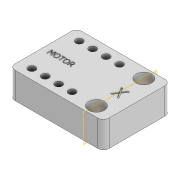
# Autodesk Inventor part: intake motor mount to xrail fixed position
Saved by Autodesk Inventor 2020 (Build 240168000, 168)
## iProperties
Created: 2020-01-10
Part Number: intake motor mount to xrail fixed position
Material: Generic
Document SubType Name: Modeling
Designer: ball
Density: 1 g/cm^3
Appearance: Default
Author: ball
Autodesk Inventor part; units mm, degrees
ref_plane "XZ Plane" through (0, 0, 0) normal (0, 1, 0) x (-1, 0, 0)
ref_plane "XY Plane" through (0, 0, 0) normal (0, 0, 1) x (1, 0, 0)
sketch "Sketch1" plane through (0, 0, 0) normal (0, 1, 0) x (-1, 0, 0)
  line L0 (-9.525, 19.05) -> (43.815, 19.05)
  line L1 (43.815, 19.05) -> (43.815, -19.05)
  line L2 (43.815, -19.05) -> (-9.525, -19.05)
  line L3 (-9.525, -19.05) -> (-9.525, 19.05)
  point P0 (0, 0)
  dimension "d0" = 53.34
  dimension "d1" = 38.1
  dimension "d3" = 9.525
  dimension "d4" = 19.05
  constraints: 8 end point, 2 parallel, 1 horizontal, 1 perpendicular
  measures "d0" distance of L1.end L2.end
  measures "d1" distance of L0.end L1.end
  measures "d3" distance from line of L3 point (0, 0)
  measures "d4" distance from line of L0 point (0, 0)
extrude "Extrusion1" add sketch "Sketch1" along normal blind 14.986
sketch "Sketch2" plane through (0, 14.986, 0) normal (0, 1, 0) x (1, 0, 0)
  line L0 (9.525, -19.05) -> (9.525, 19.05) projected
  point P0 (0, 0)
  point P1 (0, -13.4747)
  point P2 (0, 13.4747)
  dimension "d7" = 26.9494
  dimension "d9" = 9.525
  dimension "d10" = 9.525
  dimension "d11" = 13.4747
  measures "d7" distance of point (0, 13.475) point (0, -13.475)
  measures "d9" distance from line of L0 point (0, -13.475)
  measures "d10" distance from line of L0 point (0, 13.475)
  measures "d11" distance of point (0, -13.475) point (0, 0)
hole "Hole1" at (0, 14.986, 13.4747) at (0, 14.986, -13.4747) direction (0, -1, 0) diameter 4.064 end through all counterbore diameter 8.89 counterbore depth 9.0424
fillet "Fillet1" radius 3.175 4 edges at (9.525, 7.493, 19.05) (9.525, 7.493, -19.05) (-43.815, 7.493, 19.05) (-43.815, 7.493, -19.05)
sketch "Sketch5" plane through (0, 0, 0) normal (0, -1, 0) x (1, 0, 0)
  line L0 (-43.815, -15.875) -> (-43.815, 15.875) projected
  line L1 (-40.64, 19.05) -> (6.35, 19.05) projected
  line L2 (6.35, -19.05) -> (-40.64, -19.05) projected
  circle A0 centre (0, 13.4747) radius 2.032 projected
  circle A1 centre (0, -13.4747) radius 2.032 projected
  point P0 (0, 0)
  point P1 (-36.703, 13.4747)
  point P2 (-36.703, -13.4747)
  point P3 (-29.083, 13.4747)
  point P4 (-29.083, -13.4747)
  point P5 (-21.463, 13.4747)
  point P6 (-21.463, -13.4747)
  point P7 (-13.843, 13.4747)
  point P8 (-13.843, -13.4747)
  dimension "d46" = 36.703
  dimension "d47" = 36.703
  dimension "d54" = 7.62
  dimension "d59" = 26.9494
  dimension "d60" = 5.5753
  dimension "d61" = 5.5753
  constraints: 1 horizontal, 6 other
  measures "d46" distance of point (-36.703, 13.475) A0.centre
  measures "d47" distance of point (-36.703, -13.475) A1.centre
  measures "d54" distance of point (-36.703, 13.475) point (-29.083, 13.475)
  measures "d59" distance of point (-36.703, -13.475) point (-36.703, 13.475)
  measures "d60" distance from line of L1 point (-36.703, 13.475)
  measures "d61" distance from line of L2 point (-36.703, -13.475)
hole "Hole2" at (-36.703, 0, 13.4747) at (-36.703, 0, -13.4747) at (-29.083, 0, 13.4747) at (-21.463, 0, 13.4747) at (-13.843, 0, 13.4747) at (-29.083, 0, -13.4747) at (-21.463, 0, -13.4747) at (-13.843, 0, -13.4747) direction (0, 1, 0) diameter 4.064 end through all counterbore diameter 8.89 counterbore depth 6.35
sketch "Sketch6" plane through (0, 14.986, 0) normal (0, 1, 0) x (1, 0, 0)
  line L0 (-3.6028, 5.8754) -> (4.1571, 5.8754) construction
  line L1 (4.1571, 5.8754) -> (4.1571, -6.6514) construction
  line L2 (4.1571, -6.6514) -> (-3.6028, -6.6514) construction
  line L3 (-3.6028, -6.6514) -> (-3.6028, 5.8754) construction
  line L4 (-37.8576, 8.3143) -> (-28.9891, 8.3143) construction
  line L5 (-28.9891, 8.3143) -> (-28.9891, -8.4251) construction
  line L6 (-28.9891, -8.4251) -> (-37.8576, -8.4251) construction
  line L7 (-37.8576, -8.4251) -> (-37.8576, 8.3143) construction
  line L8 (-37.6075, -1.5794) -> (-38.0126, -1.5794)
  line L9 (-38.0126, -1.5794) -> (-38.0126, 1.0462)
  line L10 (-38.0126, 1.0462) -> (-38.808, -0.7396)
  line L11 (-38.808, -0.7396) -> (-39.055, -0.7396)
  line L12 (-39.055, -0.7396) -> (-39.8429, 1.0462)
  line L13 (-39.8429, 1.0462) -> (-39.8429, -1.5794)
  line L14 (-39.8429, -1.5794) -> (-40.2208, -1.5794)
  line L15 (-40.2208, -1.5794) -> (-40.2208, 1.4686)
  line L16 (-40.2208, 1.4686) -> (-39.6675, 1.4686)
  line L17 (-39.6675, 1.4686) -> (-38.9068, -0.2283)
  line L18 (-38.9068, -0.2283) -> (-38.1707, 1.4686)
  line L19 (-38.1707, 1.4686) -> (-37.6075, 1.4686)
  line L20 (-37.6075, 1.4686) -> (-37.6075, -1.5794)
  spline S0 degree 2 poles (-34.8337, 1.1203) (-34.6608, 0.9178) (-34.4682, 0.325) (-34.4682, -0.0554) knots 0 0 0 1 2 2 2
  spline S1 degree 2 poles (-34.4682, -0.0554) (-34.4682, -0.4259) (-34.6559, -1.0261) (-34.8337, -1.2287) knots 0 0 0 1 2 2 2
  spline S2 degree 2 poles (-34.8337, -1.2287) (-35.0214, -1.4411) (-35.5179, -1.6436) (-35.8168, -1.6436) knots 0 0 0 1 2 2 2
  spline S3 degree 2 poles (-35.8168, -1.6436) (-36.1255, -1.6436) (-36.6195, -1.4337) (-36.7999, -1.2287) knots 0 0 0 1 2 2 2
  spline S4 degree 2 poles (-36.7999, -1.2287) (-36.9752, -1.0261) (-37.1629, -0.4309) (-37.1629, -0.0554) knots 0 0 0 1 2 2 2
  spline S5 degree 2 poles (-37.1629, -0.0554) (-37.1629, 0.3274) (-36.9728, 0.9103) (-36.7974, 1.1203) knots 0 0 0 1 2 2 2
  spline S6 degree 2 poles (-36.7974, 1.1203) (-36.6195, 1.3228) (-36.1231, 1.5328) (-35.8168, 1.5328) knots 0 0 0 1 2 2 2
  spline S7 degree 2 poles (-35.8168, 1.5328) (-35.5056, 1.5328) (-35.0066, 1.3154) (-34.8337, 1.1203) knots 0 0 0 1 2 2 2
  spline S8 degree 2 poles (-34.8905, -0.0554) (-34.8905, 0.2459) (-35.0214, 0.7127) (-35.14, 0.8659) knots 0 0 0 1 2 2 2
  spline S9 degree 2 poles (-35.14, 0.8659) (-35.261, 1.024) (-35.6019, 1.182) (-35.8143, 1.182) knots 0 0 0 1 2 2 2
  spline S10 degree 2 poles (-35.8143, 1.182) (-36.0341, 1.182) (-36.3651, 1.0289) (-36.4911, 0.8659) knots 0 0 0 1 2 2 2
  spline S11 degree 2 poles (-36.4911, 0.8659) (-36.6121, 0.7103) (-36.7406, 0.241) (-36.7406, -0.0554) knots 0 0 0 1 2 2 2
  spline S12 degree 2 poles (-36.7406, -0.0554) (-36.7406, -0.6556) (-36.2367, -1.2929) (-35.8143, -1.2929) knots 0 0 0 1 2 2 2
  spline S13 degree 2 poles (-35.8143, -1.2929) (-35.3919, -1.2929) (-34.8905, -0.6556) (-34.8905, -0.0554) knots 0 0 0 1 2 2 2
  line L21 (-33.3122, -1.5794) -> (-33.3122, 1.1079)
  line L22 (-33.3122, 1.1079) -> (-34.3348, 1.1079)
  line L23 (-34.3348, 1.1079) -> (-34.3348, 1.4686)
  line L24 (-34.3348, 1.4686) -> (-31.8845, 1.4686)
  line L25 (-31.8845, 1.4686) -> (-31.8845, 1.1079)
  line L26 (-31.8845, 1.1079) -> (-32.9071, 1.1079)
  line L27 (-32.9071, 1.1079) -> (-32.9071, -1.5794)
  line L28 (-32.9071, -1.5794) -> (-33.3122, -1.5794)
  spline S14 degree 2 poles (-29.4194, 1.1203) (-29.2465, 0.9178) (-29.0539, 0.325) (-29.0539, -0.0554) knots 0 0 0 1 2 2 2
  spline S15 degree 2 poles (-29.0539, -0.0554) (-29.0539, -0.4259) (-29.2416, -1.0261) (-29.4194, -1.2287) knots 0 0 0 1 2 2 2
  spline S16 degree 2 poles (-29.4194, -1.2287) (-29.6072, -1.4411) (-30.1036, -1.6436) (-30.4025, -1.6436) knots 0 0 0 1 2 2 2
  spline S17 degree 2 poles (-30.4025, -1.6436) (-30.7113, -1.6436) (-31.2053, -1.4337) (-31.3856, -1.2287) knots 0 0 0 1 2 2 2
  spline S18 degree 2 poles (-31.3856, -1.2287) (-31.5609, -1.0261) (-31.7487, -0.4309) (-31.7487, -0.0554) knots 0 0 0 1 2 2 2
  spline S19 degree 2 poles (-31.7487, -0.0554) (-31.7487, 0.3274) (-31.5585, 0.9103) (-31.3831, 1.1203) knots 0 0 0 1 2 2 2
  spline S20 degree 2 poles (-31.3831, 1.1203) (-31.2053, 1.3228) (-30.7088, 1.5328) (-30.4025, 1.5328) knots 0 0 0 1 2 2 2
  spline S21 degree 2 poles (-30.4025, 1.5328) (-30.0913, 1.5328) (-29.5923, 1.3154) (-29.4194, 1.1203) knots 0 0 0 1 2 2 2
  spline S22 degree 2 poles (-29.4763, -0.0554) (-29.4763, 0.2459) (-29.6072, 0.7127) (-29.7257, 0.8659) knots 0 0 0 1 2 2 2
  spline S23 degree 2 poles (-29.7257, 0.8659) (-29.8468, 1.024) (-30.1876, 1.182) (-30.4, 1.182) knots 0 0 0 1 2 2 2
  spline S24 degree 2 poles (-30.4, 1.182) (-30.6199, 1.182) (-30.9509, 1.0289) (-31.0768, 0.8659) knots 0 0 0 1 2 2 2
  spline S25 degree 2 poles (-31.0768, 0.8659) (-31.1979, 0.7103) (-31.3263, 0.241) (-31.3263, -0.0554) knots 0 0 0 1 2 2 2
  spline S26 degree 2 poles (-31.3263, -0.0554) (-31.3263, -0.6556) (-30.8224, -1.2929) (-30.4, -1.2929) knots 0 0 0 1 2 2 2
  spline S27 degree 2 poles (-30.4, -1.2929) (-29.9777, -1.2929) (-29.4763, -0.6556) (-29.4763, -0.0554) knots 0 0 0 1 2 2 2
  line L29 (-26.2504, -1.5794) -> (-26.7765, -1.5794)
  line L30 (-26.7765, -1.5794) -> (-27.7398, -0.3667)
  line L31 (-27.7398, -0.3667) -> (-28.2042, -0.3667)
  line L32 (-28.2042, -0.3667) -> (-28.2042, -1.5794)
  line L33 (-28.2042, -1.5794) -> (-28.6093, -1.5794)
  line L34 (-28.6093, -1.5794) -> (-28.6093, 1.4686)
  line L35 (-28.6093, 1.4686) -> (-27.8238, 1.4686)
  spline S28 degree 2 poles (-27.8238, 1.4686) (-27.562, 1.4686) (-27.2088, 1.4118) (-27.0482, 1.308) knots 0 0 0 1 2 2 2
  spline S29 degree 2 poles (-27.0482, 1.308) (-26.8877, 1.2043) (-26.7024, 0.8807) (-26.7024, 0.6411) knots 0 0 0 1 2 2 2
  spline S30 degree 2 poles (-26.7024, 0.6411) (-26.7024, 0.3077) (-27.0433, -0.1443) (-27.3347, -0.253) knots 0 0 0 1 2 2 2
  line L36 (-27.3347, -0.253) -> (-26.2504, -1.5794)
  spline S31 degree 2 poles (-27.1248, 0.609) (-27.1248, 0.7424) (-27.2187, 0.9474) (-27.3175, 1.0141) knots 0 0 0 1 2 2 2
  spline S32 degree 2 poles (-27.3175, 1.0141) (-27.4039, 1.0709) (-27.6336, 1.1178) (-27.8016, 1.1178) knots 0 0 0 1 2 2 2
  line L37 (-27.8016, 1.1178) -> (-28.2042, 1.1178)
  line L38 (-28.2042, 1.1178) -> (-28.2042, -0.0283)
  line L39 (-28.2042, -0.0283) -> (-27.8485, -0.0283)
  spline S33 degree 2 poles (-27.8485, -0.0283) (-27.6731, -0.0283) (-27.394, 0.0335) (-27.2977, 0.1298) knots 0 0 0 1 2 2 2
  spline S34 degree 2 poles (-27.2977, 0.1298) (-27.2088, 0.2138) (-27.1248, 0.4509) (-27.1248, 0.609) knots 0 0 0 1 2 2 2
  line L40 (2.6755, -3.436) -> (1.7468, -3.436)
  line L41 (1.7468, -3.436) -> (0.2648, -1.0055)
  line L42 (0.2648, -1.0055) -> (-1.2469, -3.436)
  line L43 (-1.2469, -3.436) -> (-2.1212, -3.436)
  line L44 (-2.1212, -3.436) -> (-0.1798, -0.3831)
  line L45 (-0.1798, -0.3831) -> (-2.062, 2.66)
  line L46 (-2.062, 2.66) -> (-1.1332, 2.66)
  line L47 (-1.1332, 2.66) -> (0.3191, 0.274)
  line L48 (0.3191, 0.274) -> (1.8011, 2.66)
  line L49 (1.8011, 2.66) -> (2.6755, 2.66)
  line L50 (2.6755, 2.66) -> (0.7687, -0.3435)
  line L51 (0.7687, -0.3435) -> (2.6755, -3.436)
  point P0 (0, 0)
  constraints: 4 other
emboss "Emboss1" sketch "Sketch6" operation cut depth 0.635 direction (0, -1, 0)
equation "\"d4\" = 0.5 * d1"
equation "\"d9\" = d3"
equation "\"d10\" = d9"
equation "\"d11\" = 0.5 * d7"
equation "\"d47\" = d46"
body "Solid1"
